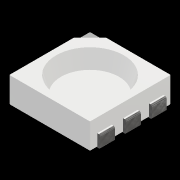
# Autodesk Inventor part: LED SMD 5050
Saved by Autodesk Inventor 2017 SP1 (Build 210196100, 196)
## iProperties
Part Number: LED SMD 5050
Material: Типовые
Document SubType Name: Modeling
Designer: Boris
Density: 1 g/cm^3
Appearance: Белый
Author: Boris
Autodesk Inventor part; units mm, degrees
ref_plane "YZ Plane" through (0, 0, 0) normal (1, 0, 0) x (0, 1, 0)
ref_plane "XZ Plane" through (0, 0, 0) normal (0, 1, 0) x (-1, 0, 0)
sketch "Эскиз1" plane through (0, 0, 0) normal (0, 0, 1) x (1, 0, 0)
  line L0 (-0.5, -0.45) -> (0.5, -0.45)
  line L1 (0.5, -0.45) -> (0.5, 0.45)
  line L2 (0.5, 0.45) -> (-0.5, 0.45)
  line L3 (-0.5, 0.45) -> (-0.5, -0.45)
  line L4 (-0.5, -0.45) -> (0.5, 0.45) construction
  line L5 (0.5, -0.45) -> (-0.5, 0.45) construction
  point P0 (0, 0)
  dimension "d0" = 1
  dimension "d1" = 0.9
  constraints: 12 end point, 2 midpoint, 2 parallel, 1 horizontal, 1 perpendicular
  measures "d0" distance of L2.end L1.end
  measures "d1" distance of L1.end L0.end
extrude "Выдавливание1" add sketch "Эскиз1" along normal blind 0.02
pattern_linear "Прямоуг.массив1" count 3 spacing 1.6 along (0, -1, 0) count 2 spacing 4.4 along (1, 0, 0) of "Выдавливание1"
sketch "Эскиз2" plane through (0, 0, 0.02) normal (0, 0, 1) x (1, 0, 0)
  line L0 (0.5, 0.45) -> (-0.5, 0.45) projected
  line L1 (-0.5, 0.45) -> (-0.5, -0.45) projected
  line L2 (3.9, -3.65) -> (4.9, -3.65) projected
  line L3 (4.9, -3.65) -> (4.9, -2.75) projected
  line L4 (4.9, -2.75) -> (3.9, -2.75) projected
  line L5 (3.9, -2.75) -> (3.9, -3.65) projected
  line L6 (3.9, -0.45) -> (4.9, -0.45) projected
  line L7 (4.9, -0.45) -> (4.9, 0.45) projected
  line L8 (4.9, 0.45) -> (3.9, 0.45) projected
  line L9 (3.9, 0.45) -> (3.9, -0.45) projected
  line L10 (-0.3, 0.9) -> (4.7, 0.9)
  line L11 (4.7, 0.9) -> (4.7, -4.1)
  line L12 (4.7, -4.1) -> (-0.3, -4.1)
  line L13 (-0.3, -4.1) -> (-0.3, 0.9)
  point P0 (0, 0)
  dimension "d10" = 5.4
  dimension "d11" = 5
  dimension "d12" = 5
  dimension "d13" = 0.2
  dimension "d14" = 4.1
  dimension "d15" = 0.45
  constraints: 8 end point, 2 parallel, 1 horizontal, 1 perpendicular
  measures "d10" distance between parallel lines of L1 L7
  measures "d11" distance of L11.end L12.end
  measures "d12" distance of L10.end L11.end
  measures "d13" distance between parallel lines of L1 L13
  measures "d14" distance from line of L2.end L8
  measures "d15" distance between parallel lines of L10 L0
extrude "Выдавливание2" add sketch "Эскиз2" along normal blind 1.6 contours L5 L4 L11 L2 | L2 L11 L12 L13 L10 L8 L9 L6 L4 L5 | L6 L9 L8 L11
sketch "Эскиз3" plane through (0, 0, 0.02) normal (0, 0, 1) x (1, 0, 0)
  line L0 (-0.3, -0.45) -> (-0.3, 0.45) projected
  line L1 (-0.3, 0.45) -> (-0.5, 0.45) projected
  line L2 (-0.5, 0.45) -> (-0.5, -0.45) projected
  line L3 (-0.5, -0.45) -> (-0.3, -0.45) projected
  line L4 (-0.3, -2.05) -> (-0.3, -1.15) projected
  line L5 (-0.3, -1.15) -> (-0.5, -1.15) projected
  line L6 (-0.5, -1.15) -> (-0.5, -2.05) projected
  line L7 (-0.5, -2.05) -> (-0.3, -2.05) projected
  line L8 (-0.5, -2.75) -> (-0.5, -3.65) projected
  line L9 (-0.3, -3.65) -> (-0.3, -2.75) projected
  line L10 (-0.3, -2.75) -> (-0.5, -2.75) projected
  line L11 (-0.5, -2.75) -> (-0.5, -3.65) projected
  line L12 (-0.5, -3.65) -> (-0.3, -3.65) projected
  line L13 (4.7, 0.45) -> (4.7, -0.45) projected
  line L14 (4.7, -0.45) -> (4.9, -0.45) projected
  line L15 (4.9, -0.45) -> (4.9, 0.45) projected
  line L16 (4.9, 0.45) -> (4.7, 0.45) projected
  line L17 (4.7, -1.15) -> (4.7, -2.05) projected
  line L18 (4.7, -2.05) -> (4.9, -2.05) projected
  line L19 (4.9, -2.05) -> (4.9, -1.15) projected
  line L20 (4.9, -1.15) -> (4.7, -1.15) projected
  line L21 (4.7, -2.75) -> (4.7, -3.65) projected
  line L22 (4.7, -3.65) -> (4.9, -3.65) projected
  line L23 (4.9, -3.65) -> (4.9, -2.75) projected
  line L24 (4.9, -2.75) -> (4.7, -2.75) projected
  point P0 (0, 0)
extrude "Выдавливание3" add sketch "Эскиз3" along normal blind 0.75
fillet "Сопряжение1" radius 0.1 12 edges at (4.9, -3.2, 0.77) (4.9, -1.6, 0.77) (4.9, 0, 0.77) (-0.5, 0, 0.77) (-0.5, -1.6, 0.77) (-0.5, -3.2, 0.77) (-0.5, -3.2, 0) (-0.5, -1.6, 0) (-0.5, 0, 0) (4.9, -3.2, 0) (4.9, -1.6, 0) (4.9, 0, 0)
fillet "Сопряжение2" radius 0.05 14 edges at (2.2, -4.1, 0.02) (4.7, -3.875, 0.02) (4.7, -2.4, 0.02) (4.7, -4.1, 0.82) (-0.3, -4.1, 0.82) (4.7, -0.8, 0.02) (4.7, 0.675, 0.02) (4.7, 0.9, 0.82) (2.2, 0.9, 0.02) (-0.3, 0.9, 0.82) (-0.3, 0.675, 0.02) (-0.3, -0.8, 0.02) (-0.3, -2.4, 0.02) (-0.3, -3.875, 0.02)
sketch "Эскиз4" plane through (0, 0, 1.62) normal (0, 0, 1) x (1, 0, 0)
  line L0 (4.65, 0.9) -> (-0.25, 0.9) projected
  line L1 (-0.3, 0.85) -> (-0.3, -4.05) projected
  line L2 (-0.3, 0.45) -> (-0.3, 0.85) projected
  line L3 (-0.3, -0.1) -> (0.7, 0.9)
  line L4 (-0.25, 0.9) -> (4.65, 0.9) projected
  arc A0 (4.7, 0.85) -> (4.65, 0.9) centre (4.65, 0.85) ccw projected
  line L5 (4.65, 0.9) -> (-0.25, 0.9) projected
  arc A1 (-0.25, 0.9) -> (-0.3, 0.85) centre (-0.25, 0.85) ccw projected
  line L6 (-0.3, 0.85) -> (-0.3, -4.05) projected
  arc A2 (-0.3, -4.05) -> (-0.25, -4.1) centre (-0.25, -4.05) ccw projected
  line L7 (-0.25, -4.1) -> (4.65, -4.1) projected
  arc A3 (4.65, -4.1) -> (4.7, -4.05) centre (4.65, -4.05) ccw projected
  line L8 (4.7, -4.05) -> (4.7, 0.85) projected
  line L9 (-0.3, -0.1) -> (-0.3, 0.9)
  line L10 (-0.3, 0.9) -> (0.7, 0.9)
  point P0 (0, 0)
  dimension "d22" = 45
  dimension "d23" = 1
  constraints: 6 end point, 3 point on line, 1 collinear
  measures "d22" angle of L0 L3
  measures "d23" distance from line of L1 L3.end
extrude "Выдавливание4" cut sketch "Эскиз4" against normal blind 0.2 contours L3 L1 A1 L0 | A1 L9 L10
ref_plane "РабПлоскость1" through (-0.25, -1.6, 1.62) normal (0, -1, 0) x (1, 0, 0)
sketch "Эскиз5" plane through (-0.25, -1.6, 1.62) normal (0, -1, 0) x (1, 0, 0)
  line L0 (4.9, -1.6) -> (0, -1.6) projected
  line L1 (2.45, -1.6) -> (2.45, 0)
  line L2 (4.9, 0) -> (0.95, 0) projected
  line L3 (2.45, -1.1766) -> (2.45, -1)
  line L4 (0.65, -1) -> (0.35, 0)
  line L5 (2.45, 0) -> (0.35, 0)
  line L6 (0.65, -1) -> (2.45, -1)
  point P0 (0.25, -1.62)
  dimension "d26" = 1.8
  dimension "d27" = 2.1
  dimension "d28" = 1
  constraints: 10 end point, 4 point on line, 1 midpoint, 1 perpendicular, 1 vertical
  measures "d26" distance from line of L1 L4.start
  measures "d27" distance from line of L4.end L1
  measures "d28" distance between parallel lines of L2 L6
revolve "Вращение1" cut sketch "Эскиз5" angle 360 about axis through (2.2, -1.6, 0.02) along (0, 0, 1)
equation "\"d13\" = -0.5 * d11 + 0.5 * d10"
equation "\"d15\" = -0.5 * d14 + 0.5 * d12"
